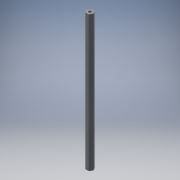
# Autodesk Inventor part: hexShaft
Saved by Autodesk Inventor 2019.4 (Build 234330000, 330)
## iProperties
Created: 2019-04-30
Part Number: hexShaft
Material: Generic
Document SubType Name: Modeling
Designer: steele
Density: 1 g/cm^3
Appearance: Default
Author: steele
Autodesk Inventor part; units mm, degrees
ref_plane "YZ Plane" through (0, 0, 0) normal (1, 0, 0) x (0, 1, 0)
ref_plane "XZ Plane" through (0, 0, 0) normal (0, 1, 0) x (-1, 0, 0)
ref_plane "XY Plane" through (0, 0, 0) normal (0, 0, 1) x (1, 0, 0)
sketch "Sketch1" plane through (0, 0, 0) normal (0, 1, 0) x (-1, 0, 0)
  line L0 (-3.9595, -6.858) -> (-7.9189, 0)
  line L1 (-7.9189, 0) -> (-3.9595, 6.858)
  line L2 (-3.9595, 6.858) -> (3.9595, 6.858)
  line L3 (3.9595, 6.858) -> (7.9189, 0)
  line L4 (7.9189, 0) -> (3.9595, -6.858)
  line L5 (3.9595, -6.858) -> (-3.9595, -6.858)
  circle A0 centre (0, 0) radius 3.175
  dimension "d0" = 13.716
  dimension "d3" = 6.35
  constraints: 12 end point, 2 coincident, 1 centre point, 1 horizontal, 13 other
  measures "d0" distance between parallel lines of L2 L5
  measures "d3" diameter of A0
extrude "Extrusion2" add sketch "Sketch1" along normal blind 304.8
body "Solid2"
